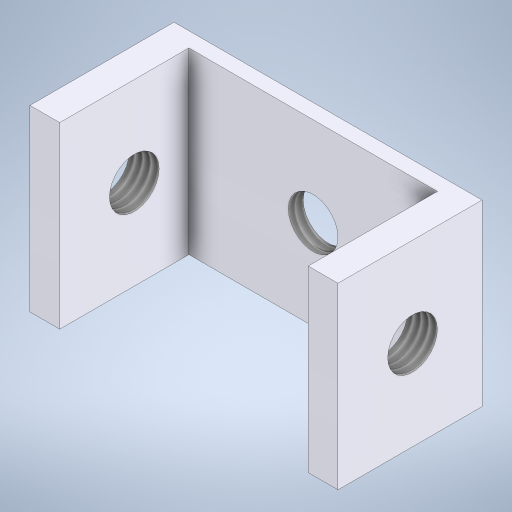
# Autodesk Inventor part: penyangga kamera 1
Saved by Autodesk Inventor 2023 (Build 270158000, 158)
## iProperties
Created: 2025-05-30
Part Number: penyangga kamera 1
Material: Generic
Document SubType Name: Modeling
Designer: ASUS
Density: 1 g/cm^3
Appearance: Default
Author: ASUS
Autodesk Inventor part; units mm, degrees
ref_plane "YZ Plane" through (0, 0, 0) normal (1, 0, 0) x (0, 1, 0)
ref_plane "XZ Plane" through (0, 0, 0) normal (0, 1, 0) x (-1, 0, 0)
ref_plane "XY Plane" through (0, 0, 0) normal (0, 0, 1) x (1, 0, 0)
sketch "Sketch1" plane through (0, 0, 0) normal (0, 0, 1) x (1, 0, 0)
  line L0 (6.9242, 30.3294) -> (37.9242, 30.3294)
  line L1 (37.9242, 30.3294) -> (37.9242, 12.3294)
  line L2 (37.9242, 12.3294) -> (6.9242, 12.3294)
  line L3 (6.9242, 12.3294) -> (6.9242, 30.3294)
  point P0 (0, 0)
  dimension "d0" = 31
  dimension "d1" = 18
  constraints: 8 end point, 2 parallel, 1 horizontal, 1 perpendicular
  measures "d0" distance of L1.end L2.end
  measures "d1" distance of L0.end L1.end
extrude "Extrusion1" add sketch "Sketch1" along normal blind 1.5
sketch "Sketch2" plane through (0, 0, 1.5) normal (0, 0, 1) x (1, 0, 0)
  line L0 (37.9242, 30.3294) -> (6.9242, 30.3294) projected
  line L1 (6.9242, 30.3294) -> (9.9242, 30.3294)
  line L2 (9.9242, 30.3294) -> (9.9242, 12.3294)
  line L3 (9.9242, 12.3294) -> (6.9242, 12.3294)
  line L4 (6.9242, 12.3294) -> (6.9242, 30.3294)
  line L5 (37.9242, 12.3294) -> (37.9242, 30.3294) projected
  line L6 (37.9242, 30.3294) -> (34.9242, 30.3294)
  line L7 (34.9242, 30.3294) -> (34.9242, 12.3294)
  line L8 (34.9242, 12.3294) -> (37.9242, 12.3294)
  line L9 (37.9242, 12.3294) -> (37.9242, 30.3294)
  point P0 (0, 0)
  dimension "d4" = 3
  dimension "d5" = 18
  dimension "d6" = 3
  dimension "d7" = 18
  constraints: 16 end point, 4 parallel, 2 horizontal, 2 perpendicular
  measures "d4" distance of L2.end L3.end
  measures "d5" distance of L1.end L2.end
  measures "d6" distance of L8.end L7.end
  measures "d7" distance of L7.end L6.end
extrude "Extrusion2" add sketch "Sketch2" along normal blind 13
sketch "Sketch3" plane through (6.9242, 12.3294, 0) normal (-1, 0, 0) x (0, 0, 1)
  line L0 (0, 18) -> (0, 0) projected
  circle A0 centre (7, 9) radius 2.5
  point P0 (0, -12.3294)
  constraints: 1 centre point
extrude "Extrusion3" cut sketch "Sketch3" against normal blind 50
sketch "Sketch4" plane through (0, 0, 1.5) normal (0, 0, 1) x (1, 0, 0)
  line L0 (37.9242, 30.3294) -> (6.9242, 30.3294) projected
  line L1 (6.9242, 12.3294) -> (37.9242, 12.3294) projected
  circle A0 centre (22.4242, 21.3294) radius 2.5
  point P0 (0, 0)
  constraints: 1 centre point
extrude "Extrusion4" cut sketch "Sketch4" against normal blind 50
thread "Thread1" size "M5x0.8" class "6H" standard "ANSI Metric M Profile" length 43.6
thread "Thread2" size "M5x0.8" class "6H" standard "ANSI Metric M Profile" length 43.6
thread "Thread3" size "M5x0.8" class "6H" standard "ANSI Metric M Profile" length 43.6
body "Solid1"
